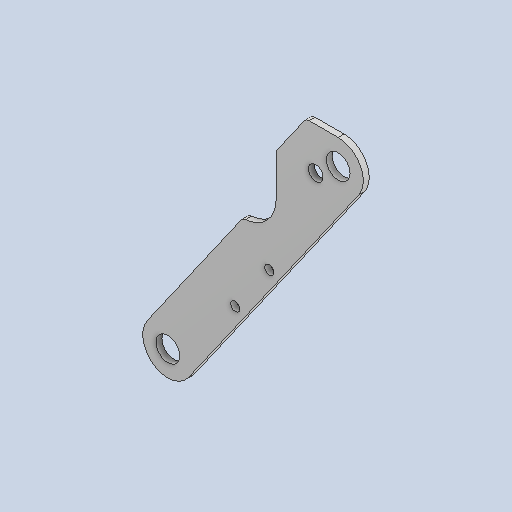
# Autodesk Inventor part: BackLink_frame
Saved by Autodesk Inventor 2022.4 (Build 264492000, 492)
## iProperties
Created: 2021-10-04
Part Number: BackLink_frame
Material: GFRP
Document SubType Name: Modeling
Designer: Masato Kubotera
Density: 1.75 g/cm^3
Appearance: 滑らか - 淡い灰色
Description: GFRP T2
Mass: 6.44398 g
Surface Area: 43.7409 cm^2
Volume: 3.68228 cm^3
Author: Masato Kubotera
Autodesk Inventor part; units mm, degrees
ref_plane "YZ Plane" through (0, 0, 0) normal (1, 0, 0) x (0, 1, 0)
ref_plane "XZ Plane" through (0, 0, 0) normal (0, 1, 0) x (-1, 0, 0)
ref_plane "XY Plane" through (0, 0, 0) normal (0, 0, 1) x (1, 0, 0)
derived "Link_basis.ipt"
sketch "スケッチ1" plane through (0, 0, 0) normal (0, 0, 1) x (1, 0, 0)
  circle A0 centre (0, 0) radius 6
  circle A1 centre (-57.3576, -81.9152) radius 4
  arc A2 (-64.3015, -81.0305) -> (-57.3576, -88.9152) centre (-57.3576, -81.9152) ccw
  arc A3 (-0.1434, -10.9991) -> (-4.8354, 9.8802) centre (0, 0) ccw
  line L0 (-58.3761, -41.5269) -> (-32.5651, -4.6651) construction
  line L1 (-32.5651, -4.6651) -> (-28.4694, -7.533) construction
  line L2 (-28.4694, -7.533) -> (-54.2803, -44.3948) construction
  line L3 (-54.2803, -44.3948) -> (-58.3761, -41.5269) construction
  line L4 (-58.3761, -41.5269) -> (-28.4694, -7.533) construction
  line L5 (-32.5651, -4.6651) -> (-54.2803, -44.3948) construction
  line L6 (-56.3282, -42.9609) -> (-30.5172, -6.099) construction
  circle A4 centre (-54.8942, -40.913) radius 1.55
  circle A5 centre (-43.4227, -24.5299) radius 1.55
  line L7 (-45.4706, -23.096) -> (-41.3748, -25.9639) construction
  circle A6 centre (-31.9512, -8.1469) radius 1.55
  line L8 (-59.1952, -40.9534) -> (-33.3843, -4.0915)
  line L9 (-33.3843, -4.0915) -> (-4.8354, 9.8802)
  line L10 (-59.1952, -40.9534) -> (-64.3015, -81.0305)
  line L11 (-32.3614, -57.0111) -> (-0.1434, -10.9991)
  line L12 (0, 0) -> (32, 0) construction
  line L13 (32, 0) -> (32, 20) construction
  circle A7 centre (32, 20) radius 4
  arc A8 (38.9218, 15.1533) -> (32, 28.45) centre (32, 20) ccw
  line L14 (32, 20) -> (32, 37) construction
  circle A9 centre (32, 37) radius 4 construction
  circle A10 centre (32, 37) radius 8.45 construction
  line L15 (-57.3576, -81.9152) -> (0, 0) construction
  circle A11 centre (0, 0) radius 8.5 construction
  line L16 (0, 0) -> (4.8754, 6.9628) construction
  circle A12 centre (4.8754, 6.9628) radius 1.35
  circle A13 centre (32, 20) radius 7 construction
  arc A14 (-64.3015, -81.0305) -> (-53.3426, -76.1811) centre (-57.3576, -81.9152) ccw construction
  line L17 (-51.6236, -85.9302) -> (-33.7808, -60.4482)
  line L18 (38.9218, 15.1533) -> (-18.4358, -66.7619)
  line L19 (32, 20) -> (-25.3576, -61.9152) construction
  circle A15 centre (-25.3576, -61.9152) radius 4
  circle A16 centre (-25.3576, -61.9152) radius 8 construction
  arc A17 (-0.0917, -11.0996) -> (11.1, 0) centre (0, 0) ccw
  line L20 (25.0782, 24.8467) -> (10.3989, 3.8825) construction
  line L21 (-0.0917, -11.0996) -> (-32.2795, -57.0685)
  arc A18 (-32.2795, -57.0685) -> (-18.4358, -66.7619) centre (-25.3576, -61.9152) ccw
  arc A19 (-32.3614, -57.0111) -> (-32.5799, -66.4914) centre (-25.3576, -61.9152) ccw
  line L22 (-6.9628, 4.8754) -> (0, 0) construction
  circle A20 centre (-6.9628, 4.8754) radius 1.35
  circle A21 centre (-4.8754, -6.9628) radius 1.35
  circle A22 centre (6.9628, -4.8754) radius 1.35
  line L23 (-6.1434, -38.7459) -> (8.196, -18.2671) construction
  line L24 (8.196, -18.2671) -> (12.2917, -21.135) construction
  line L25 (12.2917, -21.135) -> (-2.0477, -41.6138) construction
  line L26 (-2.0477, -41.6138) -> (-6.1434, -38.7459) construction
  line L27 (-6.1434, -38.7459) -> (12.2917, -21.135) construction
  line L28 (8.196, -18.2671) -> (-2.0477, -41.6138) construction
  line L29 (10.2439, -19.701) -> (-4.0955, -40.1798) construction
  line L30 (1.0263, -28.5065) -> (5.122, -31.3744) construction
  circle A23 centre (8.8099, -21.7489) radius 1.55
  circle A24 centre (-2.6616, -38.132) radius 1.55
  line L31 (7.185, 8.4608) -> (11.1, 14.052)
  line L32 (32, 28.45) -> (21.1816, 28.45)
  arc A25 (32, 28.45) -> (25.0782, 24.8467) centre (32, 20) ccw construction
  line L33 (-32.5799, -66.4914) -> (-48.2812, -88.9152)
  line L34 (-57.3576, -88.9152) -> (-48.2812, -88.9152)
  arc A26 (-57.3576, -88.9152) -> (-51.6236, -85.9302) centre (-57.3576, -81.9152) ccw construction
  circle A27 centre (24.4425, 14.315) radius 2.4571
  line L35 (20.5285, 3.617) -> (-5.6844, 21.9714) construction
  line L36 (-5.6844, 21.9714) -> (15.7649, 3.9734) construction
  line L37 (15.7649, 3.9734) -> (24.4425, 14.315) construction
  line L38 (15.7649, 3.9734) -> (7.0872, -6.3682)
  arc A28 (6.7608, -8.8035) -> (9.4738, -5.7842) centre (7.0872, -6.3682) ccw
  line L39 (11.1, 0) -> (11.1, 14.052)
  line L40 (11.1, 14.052) -> (21.1816, 28.45)
  arc A29 (11.1, 0) -> (7.185, 8.4608) centre (0, 0) ccw construction
  point P0 (3.0742, -29.9404)
  dimension "d12" = 4.9141
  dimension "d15" = 32
  dimension "d16" = 20
  dimension "d17" = 20
  dimension "d18" = 32
  dimension "d22" = 28
  dimension "d23" = 5
  dimension "d24" = 13.5
  dimension "d25" = 13.5
  dimension "d27" = 2.4571
  measures "d12" diameter of A27
  measures "d15" distance of L35.start L35.end
  measures "d16" distance of L35.start L13.end
  measures "d17" distance of L12.end L13.end
  measures "d18" distance of L12.start L12.end
  measures "d22" distance of L35.end L36.end
  measures "d23" angle of L36 L35
  measures "d24" distance of L36.end L37.end
  measures "d25" distance of L36.end L38.end
  measures "d27" radius of A28
extrude "押し出し1" add sketch "スケッチ1" along normal blind 2 contours L18 A18 L21 A17 A28 L39 L40 L32 A8 | A17 A28
fillet "フィレット1" radius 2 3 edges at (-0.0917, -11.0996, 1) (21.1816, 28.45, 1) (11.1, 14.052, 1)
equation "\"d15\" = d18"
equation "\"d16\" = d17"
equation "\"d25\" = d24"
equation "\"d27\" = 0.5 * d12"
